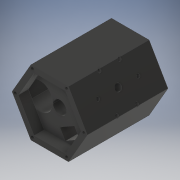
# Autodesk Inventor part: TA02
Saved by Autodesk Inventor 2017 (Build 210142000, 142)
## iProperties
Created: 2018-10-09
Part Number: TA02
Material: ABS Plastic
Document SubType Name: Modeling
Designer: Zach
Density: 1.06 g/cm^3
Appearance: Smooth - Black
Author: Zach
Autodesk Inventor part; units mm, degrees
ref_plane "YZ Plane" through (0, 0, 0) normal (1, 0, 0) x (0, 1, 0)
ref_plane "XZ Plane" through (0, 0, 0) normal (0, 1, 0) x (-1, 0, 0)
ref_plane "XY Plane" through (0, 0, 0) normal (0, 0, 1) x (1, 0, 0)
sketch "Sketch1" plane through (0, 0, 0) normal (0, 0, 1) x (1, 0, 0)
  circle A0 centre (0, 0) radius 56
  circle A1 centre (0, 0) radius 10
  circle A2 centre (-30, 0) radius 4
  line L0 (-39, 9) -> (-21, 9) construction
  line L1 (-21, 9) -> (-21, -9) construction
  line L2 (-21, -9) -> (-39, -9) construction
  line L3 (-39, -9) -> (-39, 9) construction
  circle A3 centre (-39, 9) radius 2
  circle A4 centre (-21, 9) radius 2
  circle A5 centre (-21, -9) radius 2
  circle A6 centre (-39, -9) radius 2
  circle A7 centre (15, 25.9808) radius 3.5
  line L4 (0, 0) -> (-30, 0) construction
  line L5 (0, 0) -> (15, 25.9808) construction
  line L6 (0, 0) -> (15, -25.9808) construction
  circle A8 centre (15, -25.9808) radius 3.5
  point P0 (-39, 0)
  point P1 (-30, 9)
  dimension "d0" = 112
  dimension "d1" = 20
  dimension "d2" = 8
  dimension "d3" = 30
  dimension "d4" = 18
  dimension "d5" = 18
  dimension "d6" = 4
  dimension "d7" = 4
  dimension "d8" = 4
  dimension "d9" = 4
  dimension "d10" = 7
  dimension "d11" = 30
  dimension "d12" = 120
  dimension "d13" = 30
  dimension "d14" = 7
  dimension "d15" = 120
  constraints: 14 end point, 9 centre point, 8 coincident, 2 horizontal, 2 horizontal alignment, 2 midpoint, 2 parallel, 1 perpendicular, 1 vertical alignment
  measures "d0" diameter of A0
  measures "d1" diameter of A1
  measures "d2" diameter of A2
  measures "d3" distance of L4.end point (0, 0)
  measures "d4" distance of L1.end L2.end
  measures "d5" distance of L0.end L1.end
  measures "d6" diameter of A3
  measures "d7" diameter of A4
  measures "d8" diameter of A5
  measures "d9" diameter of A6
  measures "d10" diameter of A7
  measures "d11" distance of L5.start L5.end
  measures "d12" angle of L5 L4
  measures "d13" distance of L5.start L6.end
  measures "d14" diameter of A8
  measures "d15" angle of L4 L6
extrude "Extrusion1" add sketch "Sketch1" along normal blind 5
sketch "Sketch2" plane through (0, 0, 5) normal (0, 0, 1) x (1, 0, 0)
  circle A0 centre (0, 0) radius 56 projected
  circle A1 centre (0, 0) radius 47
  dimension "d18" = 9
  constraints: 1 centre point, 1 coincident
  measures "d18" radial gap between concentric circles of A0 A1
extrude "Extrusion2" add sketch "Sketch2" along normal blind 115
sketch "Sketch3" plane through (0, 0, 5) normal (0, 0, 1) x (1, 0, 0)
  circle A0 centre (-30, 0) radius 4 projected
  circle A1 centre (0, 0) radius 10 projected
  circle A2 centre (15, 25.9808) radius 3.5 projected
  circle A3 centre (15, -25.9808) radius 3.5 projected
  circle A4 centre (-30, 0) radius 20
  line L0 (21.8253, 12.8026) -> (0.1747, 25.3026)
  line L1 (0.1747, 25.3026) -> (8.1747, 39.159)
  line L2 (8.1747, 39.159) -> (29.8253, 26.659)
  line L3 (29.8253, 26.659) -> (21.8253, 12.8026)
  line L4 (21.8253, 12.8026) -> (8.1747, 39.159) construction
  line L5 (0.1747, 25.3026) -> (29.8253, 26.659) construction
  line L6 (0, 0) -> (-30, 0) construction
  line L7 (0.1747, -25.3026) -> (21.8253, -12.8026)
  line L8 (21.8253, -12.8026) -> (29.8253, -26.659)
  line L9 (29.8253, -26.659) -> (8.1747, -39.159)
  line L10 (8.1747, -39.159) -> (0.1747, -25.3026)
  circle A5 centre (0, 0) radius 47 projected
  dimension "d21" = 40
  dimension "d23" = 120
  dimension "d24" = 16
  dimension "d25" = 25
  dimension "d28" = 120
  constraints: 22 end point, 2 midpoint, 2 parallel, 1 centre point, 1 coincident, 1 horizontal, 1 perpendicular, 9 other
  measures "d21" diameter of A4
  measures "d23" angle of L6 L1
  measures "d24" distance of L0.end L1.end
  measures "d25" distance of L1.end L2.end
extrude "Extrusion3" add sketch "Sketch3" along normal blind 100 contours A4 A5 picked at (30.2169, 0)
sketch "Sketch6" plane through (-30, 0, 5) normal (0, 0, 1) x (-0.9374167, 0.3482097, 0)
  circle A0 centre (0, 0) radius 4 projected
  circle A1 centre (0, 0) radius 16.5
  circle A2 centre (0, 0) radius 20 projected
  point P0 (-28.1225, -10.4463)
  point P1 (-18.7483, -6.9642)
  dimension "d46" = 33
  constraints: 1 centre point, 1 coincident, 1 other
  measures "d46" diameter of A1
extrude "Extrusion6" add sketch "Sketch6" along normal blind 40 contours A2
sketch "Sketch14" plane through (0, 0, 0) normal (0, 0, -1) x (-1, 0, 0)
  circle A0 centre (0, 0) radius 10 projected
  line L0 (-56, 0) -> (-28, 48.4974)
  line L1 (-28, 48.4974) -> (28, 48.4974)
  line L2 (28, 48.4974) -> (56, 0)
  line L3 (56, 0) -> (28, -48.4974)
  line L4 (28, -48.4974) -> (-28, -48.4974)
  line L5 (-28, -48.4974) -> (-56, 0)
  circle A1 centre (0, 0) radius 56 projected
  constraints: 12 end point, 2 horizontal alignment, 1 coincident, 14 other
extrude "Extrusion12" cut sketch "Sketch14" against normal through all contours A1 L0 | L5 A1 | A1 L1 | L4 A1 | A1 L2 | L3 A1
sketch "Sketch15" plane through (0, 0, 120) normal (0, 0, 1) x (1, 0, 0)
  line L0 (-28, -48.4974) -> (28, -48.4974) projected
  line L1 (-56, 0) -> (-28, -48.4974) projected
  line L2 (-28, 48.4974) -> (-56, 0) projected
  line L3 (28, 48.4974) -> (-28, 48.4974) projected
  line L4 (56, 0) -> (28, 48.4974) projected
  line L5 (28, -48.4974) -> (56, 0) projected
  line L6 (-23.3812, -40.4974) -> (23.3812, -40.4974)
  line L7 (23.3812, -40.4974) -> (46.7624, 0)
  line L8 (46.7624, 0) -> (23.3812, 40.4974)
  line L9 (23.3812, 40.4974) -> (-23.3812, 40.4974)
  line L10 (-23.3812, 40.4974) -> (-46.7624, 0)
  line L11 (-46.7624, 0) -> (-23.3812, -40.4974)
  point P0 (0, 0)
  dimension "d80" = 8
  constraints: 12 end point, 5 other
  measures "d80" distance between parallel lines of L1 L11
extrude "Extrusion13" add sketch "Sketch15" against normal blind 15
sketch "Sketch16" plane through (0, 0, 120) normal (0, 0, 1) x (1, 0, 0)
  circle A0 centre (-51, 0) radius 2.5
  line L0 (-56, 0) -> (-28, 48.4974) projected
  circle A1 centre (-25.5, -44.1673) radius 2.5
  circle A2 centre (25.5, -44.1673) radius 2.5
  circle A3 centre (51, 0) radius 2.5
  circle A4 centre (25.5, 44.1673) radius 2.5
  circle A5 centre (-25.5, 44.1673) radius 2.5
  point P0 (0, 0)
  dimension "d83" = 5
  dimension "d90" = 5
  dimension "d93" = 360
  constraints: 6 centre point, 1 coincident, 1 horizontal alignment, 13 other
  measures "d83" diameter of A0
  measures "d90" distance of L0.start A0.centre
extrude "Extrusion14" cut sketch "Sketch16" against normal blind 50
sketch "Sketch17" plane through (56, 0, 120) normal (0.8660254, 0.5, 0) x (0, 0, -1)
  line L0 (120, 84) -> (0, 84) projected
  circle A0 centre (60, 28) radius 5
  line L1 (0, 0) -> (0, 56) projected
  circle A1 centre (90, 28) radius 2.5
  circle A2 centre (75, 53.9808) radius 2.5
  circle A3 centre (45, 53.9808) radius 2.5
  circle A4 centre (30, 28) radius 2.5
  circle A5 centre (45, 2.0192) radius 2.5
  circle A6 centre (75, 2.0192) radius 2.5
  point P0 (120, 28)
  point P1 (60, 84)
  point P2 (0, 28)
  dimension "d95" = 10
  dimension "d96" = 5
  dimension "d97" = 30
  dimension "d100" = 360
  constraints: 7 centre point, 2 horizontal alignment, 2 midpoint, 1 vertical alignment, 13 other
  measures "d95" diameter of A0
  measures "d96" diameter of A1
  measures "d97" distance of A1.centre A0.centre
extrude "Extrusion15" cut sketch "Sketch17" against normal blind 25
equation "\"d3\" = d11"
equation "\"d13\" = d11"
body "Solid1"
